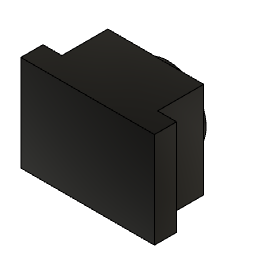
Taste_OnOff_v56 (Autodesk Fusion 360 design; units mm, degrees)
Autodesk Fusion 360 part; units mm, degrees
sketch "Skizze1" plane through (0, 0, 0) normal (0, 0, 1) x (1, 0, 0)
  line L0 (-3.8, 1.825) -> (3.8, 1.825)
  line L1 (3.8, 1.825) -> (3.8, -1.825)
  line L2 (-3.8, -1.825) -> (-3.8, 1.825)
  line L3 (-3.8, 1.825) -> (3.8, -1.825) construction
  line L4 (3.8, 1.825) -> (-3.8, -1.825) construction
  line L5 (5.3, -3.575) -> (-5.3, -3.575)
  line L6 (-5.3, -3.575) -> (-5.3, -1.825)
  line L7 (5.3, -1.825) -> (5.3, -3.575)
  line L8 (-5.3, -1.825) -> (-3.8, -1.825)
  line L9 (3.8, -1.825) -> (5.3, -1.825)
  dimension "d880" = 7.6
  dimension "d881" = 1.75
  dimension "d882" = 3.65
  dimension "d883" = 1.5
  constraint horizontal L0
  constraint perpendicular L0 L1
  constraint parallel L1 L2
  constraint coincident L3 origin
  constraint coincident L4 origin
  constraint horizontal L5
  constraint vertical L6
  constraint horizontal L8
  constraint vertical L7
  constraint horizontal L2.start L6.end
  constraint collinear L8 L9
  constraint equal L8 L9
  measures "d880" distance of L0.start L0.end
  measures "d881" distance of L5.end L6.end
  measures "d882" distance of L0.start L2.start
  measures "d883" distance of L1.end L7.start
extrude "Extrusion1" add sketch "Skizze1" along normal blind 7.6
sketch "Skizze2" plane through (0, 1.825, 0) normal (0, 1, 0) x (-1, 0, 0)
  line L0 (-3.8, 0) -> (3.8, 0)
  line L1 (3.8, 0) -> (3.8, 7.6)
  line L2 (3.8, 7.6) -> (-3.8, 7.6)
  line L3 (-3.8, 7.6) -> (-3.8, 0)
  line L4 (3.8, 7.6) -> (-3.8, 0) construction
  arc A0 (1.6, 5) -> (2.4, 5.6) centre (2, 5.3) ccw
  arc A1 (2.4, 2) -> (1.6, 2.6) centre (2, 2.3) ccw
  arc A2 (2.4, 5.6) -> (2.4, 2) centre (0, 3.8) ccw
  arc A3 (1.6, 5) -> (1.6, 2.6) centre (0, 3.8) ccw
  line L5 (2.8, 4.3) -> (0.5, 4.3)
  arc A4 (0.5, 4.3) -> (0.5, 3.3) centre (0.5, 3.8) ccw
  line L6 (0.5, 3.3) -> (2.8, 3.3)
  arc A5 (2.8, 3.3) -> (2.8, 4.3) centre (2.8, 3.8) ccw
  line L7 (2.8, 3.8) -> (0.5, 3.8) construction
  point P0 (0, 3.8)
  dimension "d906" = 1
  dimension "d907" = 6
  dimension "d908" = 1
  dimension "d909" = 0.5
  dimension "d910" = 1
  dimension "d911" = 1.5
  constraint coincident L1.end L2.start
  constraint coincident L0.start L3.end
  constraint midpoint L4 P0
  constraint coincident P0 A2.centre
  constraint tangent A0 A3
  constraint tangent A0 A2
  constraint tangent A1 A3
  constraint tangent A1 A2
  constraint vertical A0.centre A1.centre
  constraint tangent L5 A4
  constraint tangent A4 L6
  constraint parallel L5 L6
  constraint tangent L6 A5
  constraint tangent L5 A5
  constraint horizontal L7
  constraint horizontal P0 A4.centre
  measures "d906" distance of A2 A3
  measures "d907" diameter of A2
  measures "d908" distance of L5 L6
  measures "d909" distance of P0 A4.centre
  measures "d910" distance of L1 A5.centre
  measures "d911" distance of A0.centre L7
extrude "Extrusion2" add sketch "Skizze2" along normal blind 1 contours A0 A1 A2 A3 | L5 A4 L6 A5
equation "d908 = d906"
equation "d910 = d908 / 2 + 0.5 mm"
named bodies: "Taste_OnOff"
